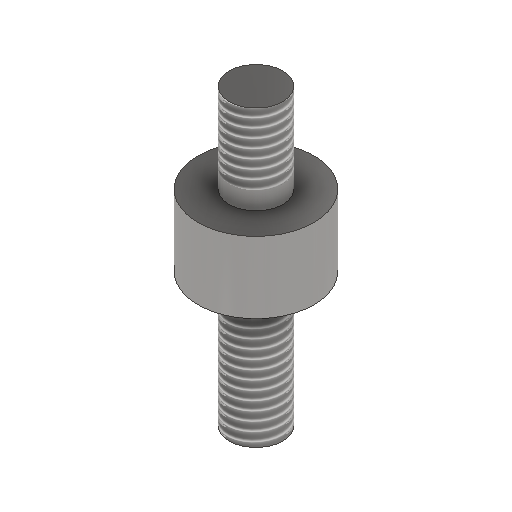
# Autodesk Inventor part: sensor_tension
Saved by Autodesk Inventor 2026.1 (Build 301233000, 233)
## iProperties
Created: 2025-10-01
Part Number: sensor_tension
Material: Genérico
Document SubType Name: Modeling
Designer: gianm
Density: 1 g/cm^3
Appearance: Acero - Pulido
Author: gianm
Autodesk Inventor part; units mm, degrees
ref_plane "YZ Plane" through (0, 0, 0) normal (1, 0, 0) x (0, 1, 0)
ref_plane "XZ Plane" through (0, 0, 0) normal (0, 1, 0) x (-1, 0, 0)
ref_plane "XY Plane" through (0, 0, 0) normal (0, 0, 1) x (1, 0, 0)
sketch "Boceto1" plane through (0, 0, 0) normal (0, 0, 1) x (1, 0, 0)
  line L0 (0, 33) -> (-3, 33)
  line L1 (-3, 33) -> (-3, 23)
  line L2 (-3, 23) -> (-6.5, 23)
  line L3 (-6.5, 23) -> (-6.5, 15)
  line L4 (-6.5, 15) -> (-3, 15)
  line L5 (0, 0) -> (-3, 0)
  line L6 (0, 33) -> (0, 0)
  line L7 (-3, 0) -> (-3, 13)
  arc A0 (-3, 13) -> (-3, 15) centre (-3, 14) ccw
  line L8 (-3, 14) -> (-3, 13) construction
  dimension "d0" = 33
  dimension "d2" = 3
  dimension "d3" = 3
  dimension "d6" = 6.5
  dimension "d7" = 13
  dimension "d8" = 10
  dimension "d9" = 15
  constraints: 18 end point, 4 vertical, 3 perpendicular, 2 horizontal, 2 point on circle, 1 centre point, 1 point on line
  measures "d0" distance of L5.start L0.start
  measures "d2" distance of L0.start L0.end
  measures "d3" distance of L5.start L5.end
  measures "d6" distance between parallel lines of L6 L3
  measures "d7" distance of L5.end L7.end
  measures "d8" vertical distance of L2.end L0.end
  measures "d9" vertical distance of L5.end L3.end
revolve "Revolución1" add sketch "Boceto1" angle 360 about axis through (0, 33, 0) along (0, -1, 0)
thread "Rosca1" size "M6x1" class "6g" standard "ANSI Metric M Profile" length 13
thread "Rosca2" size "M6x1" class "6g" standard "ANSI Metric M Profile" length 8
